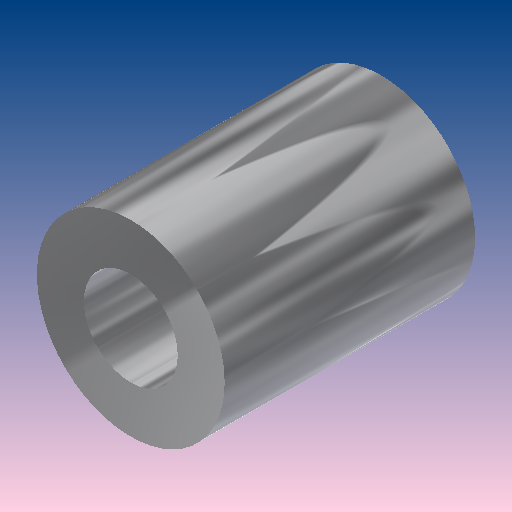
# Autodesk Inventor part: スペーサ　m3-l8
Saved by Autodesk Inventor 2019 (Build 230136000, 136)
## iProperties
Created: 2017-03-24
Part Number: スペーサ　m3-l8
Material: アルミニウム 2014-T4
Document SubType Name: Modeling
Designer: 大空
Density: 2.8 g/cm^3
Appearance: サテン
Mass: 0.475009 g
Surface Area: 2.68606 cm^2
Volume: 0.169646 cm^3
Author: 大空
Autodesk Inventor part; units mm, degrees
ref_plane "YZ Plane" through (0, 0, 0) normal (1, 0, 0) x (0, 1, 0)
ref_plane "XZ Plane" through (0, 0, 0) normal (0, 1, 0) x (-1, 0, 0)
ref_plane "XY Plane" through (0, 0, 0) normal (0, 0, 1) x (1, 0, 0)
sketch "スケッチ1" plane through (0, 0, 0) normal (0, 0, 1) x (1, 0, 0)
  circle A0 centre (0, 0) radius 1.5
  circle A1 centre (0, 0) radius 3
  dimension "d0" = 3
  dimension "d1" = 6
  constraints: 2 centre point, 2 coincident
  measures "d0" diameter of A0
  measures "d1" diameter of A1
extrude "押し出し1" add sketch "スケッチ1" along normal blind 8
